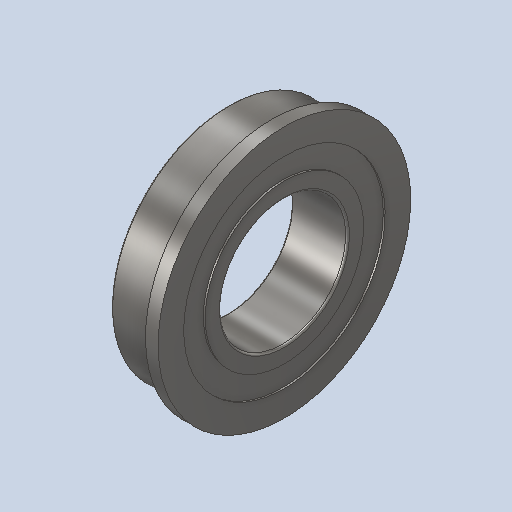
# Autodesk Inventor part: C-FL6904ZZ_CPY
Saved by Autodesk Inventor 2024 (Build 280153000, 153)
## iProperties
Created: 2023-08-11
Part Number: C-FL6904ZZ_CPY
Material: ステンレス鋼
Catalog Web Link: www.cadenas.de
Description: C-FL6900ZZ, C-FL6901ZZ, C-FL6902ZZ, C-FL6903ZZ, C-FL6904ZZ, C-FL6905ZZ-C-VALUE Medium Accuracy Small Deep Groove Ball Bearings with Flange - Double Shielded - C-FL6900ZZ
Vendor: MISUMI
Document SubType Name: Modeling
Designer: zegi
Manufacturer: MISUMI
Stock Number: 2
Mass: 56.1998 g
Surface Area: 35.9178 cm^2
Volume: 7.02498 cm^3
Density: 8 g/cm^3
Appearance: 半つや出し
Category: PARTsolutions
Company: MISUMI
Title: C-FL6904ZZ
Author: Cadenas PARTsolutions
Comments: C-VALUE Medium Accuracy Small Deep Groove Ball Bearings with Flange - Double Shielded - C-FL6900ZZ
PSOL_IDENT_0: {$CADENAS_DATA/23d-libs/misumi/metric/12_bearing_holders/c_fl6900zz.prj},225 {VTYP=3D},{NB=C-FL6904Z
PSOL_IDENT_1: Z},{LINA=C-FL6904ZZ},{NN=C-FL6900ZZ, C-FL6901ZZ, C-FL6902ZZ, C-FL6903ZZ, C-FL6904ZZ, C-FL6905ZZ},{DA
PSOL_IDENT_2: TE=29.05.2023 02:13:13},{GEOMDATE=28.10.2019 02:50:16},{VERSION=},{LINEID=990},{WBVAR=},{WBNUMERIC=}
PSOL_IDENT_3: {NB=C-FL6904ZZ},{LINA=C-FL6904ZZ},{KT=DUMMY},{PN=C-FL6904ZZ},{TS=C-FL6904ZZ},{DD=20},{D=37},{B=9},
PSOL_IDENT_4: {D1=40.0},{C=2.0},{RR=0.3},{DD1=25.10},{B1=0.30},{D2=31.9}
NB: C-FL6904ZZ
NN: C-FL6900ZZ, C-FL6901ZZ, C-FL6902ZZ, C-FL6903ZZ, C-FL6904ZZ, C-FL6905ZZ
NT: C-VALUE Medium Accuracy Small Deep Groove Ball Bearings with Flange - Double Shielded - C-FL6900ZZ
NBSYN: $PN.
LINA: C-FL6904ZZ
CATALOG: Misumi
PN: C-FL6904ZZ
TS: C-FL6904ZZ
DD: 20
D: 37
B: 9
D1: 40
C: 2
RR: 0.3
SUPPLIER: MISUMI
ARTICLENO: C-FL6904ZZ
BOMINFO: C-FL6904ZZ
CREATOR: CADENAS GmbH
Autodesk Inventor part; units mm, degrees
ref_plane "YZ Plane" through (0, 0, 0) normal (1, 0, 0) x (0, 1, 0)
ref_plane "XZ Plane" through (0, 0, 0) normal (0, 1, 0) x (-1, 0, 0)
ref_plane "XY Plane" through (0, 0, 0) normal (0, 0, 1) x (1, 0, 0)
sketch "_____1" plane through (0, 0, 0) normal (0, 0, 1) x (1, 0, 0)
  line L0 (50, 0) -> (-50, 0)
  line L1 (-4.5, 0) -> (-4.5, 12.55)
  line L2 (-4.5, 12.55) -> (-4.2, 12.55)
  line L3 (-4.2, 12.55) -> (-4.2, 15.95)
  line L4 (-4.2, 15.95) -> (-4.5, 15.95)
  line L5 (-4.5, 15.95) -> (-4.5, 18.2)
  arc A0 (-4.2, 18.5) -> (-4.5, 18.2) centre (-4.2, 18.2) ccw
  line L6 (-4.2, 18.5) -> (2.5, 18.5)
  line L7 (2.5, 18.5) -> (2.5, 20)
  line L8 (2.5, 20) -> (4.5, 20)
  line L9 (4.5, 20) -> (4.5, 15.95)
  line L10 (4.5, 15.95) -> (4.2, 15.95)
  line L11 (4.2, 15.95) -> (4.2, 12.55)
  line L12 (4.2, 12.55) -> (4.5, 12.55)
  line L13 (4.5, 12.55) -> (4.5, 0)
  line L14 (4.5, 0) -> (-4.5, 0)
  constraints: 30 end point, 2 point on circle, 1 centre point
revolve "Revolution1" add sketch "_____1" angle 360 about axis through (50, 0, 0) along (1, 0, 0)
sketch "_____2" plane through (0, 0, 0) normal (0, 0, 1) x (1, 0, 0)
  line L0 (50, 0) -> (-50, 0)
  line L1 (-4.5, 0) -> (-4.5, 10.3)
  arc A0 (-4.5, 10.3) -> (-4.2, 10) centre (-4.2, 10.3) ccw
  line L2 (-4.2, 10) -> (4.2, 10)
  arc A1 (4.2, 10) -> (4.5, 10.3) centre (4.2, 10.3) ccw
  line L3 (4.5, 10.3) -> (4.5, 0)
  line L4 (4.5, 0) -> (-4.5, 0)
  constraints: 10 end point, 4 point on circle, 2 centre point
revolve "Revolution2" cut sketch "_____2" angle 360 about axis through (50, 0, 0) along (1, 0, 0)
body "Solid1"
